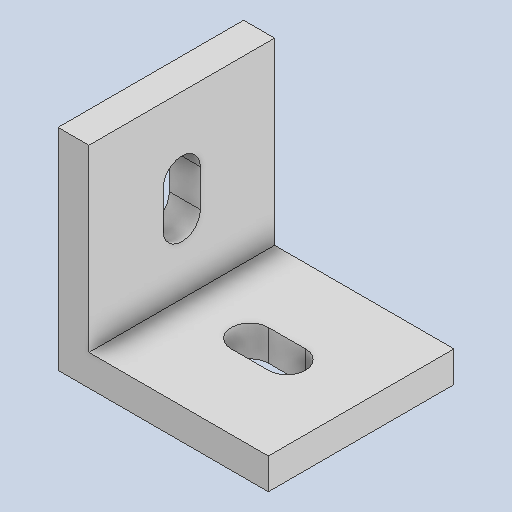
# Autodesk Inventor part: L
Saved by Autodesk Inventor 2025 (Build 290162000, 162)
## iProperties
Created: 2025-09-03
Part Number: L
Material: Generic
Document SubType Name: Modeling
Designer: Pravoslav
Density: 1 g/cm^3
Appearance: Default
Author: Pravoslav
Autodesk Inventor part; units mm, degrees
ref_plane "YZ Plane" through (0, 0, 0) normal (1, 0, 0) x (0, 1, 0)
ref_plane "XZ Plane" through (0, 0, 0) normal (0, 1, 0) x (-1, 0, 0)
ref_plane "XY Plane" through (0, 0, 0) normal (0, 0, 1) x (1, 0, 0)
sketch "Sketch1" plane through (0, 0, 0) normal (0, 1, 0) x (-1, 0, 0)
  line L0 (17, 15) -> (-17, 15)
  line L1 (-17, 15) -> (-17, -15)
  line L2 (-17, -15) -> (17, -15)
  line L3 (17, -15) -> (17, 15)
  line L4 (17, 15) -> (-17, -15) construction
  line L5 (-17, 15) -> (17, -15) construction
  circle A0 centre (-5, 0) radius 3
  circle A1 centre (1, 0) radius 3
  line L6 (1, 3) -> (-5, 3)
  line L7 (1, -3) -> (-5, -3)
  point P0 (0, 0)
  dimension "d0" = 34
  dimension "d1" = 30
  dimension "d2" = 6
  dimension "d3" = 12
  dimension "d4" = 6
  dimension "d5" = 18
  constraints: 16 end point, 4 point on circle, 3 parallel, 2 centre point, 2 horizontal, 2 midpoint, 1 perpendicular, 1 tangent
  measures "d0" distance of L2.end L1.end
  measures "d1" distance of L1.end L0.end
  measures "d2" diameter of A0
  measures "d3" distance from line of L1 A0.centre
  measures "d4" diameter of A1
  measures "d5" distance from line of L1 A1.centre
extrude "Extrusion1" add sketch "Sketch1" along normal blind 5
sketch "Sketch2" plane through (-17, 0, -15) normal (-1, 0, 0) x (0, 0, 1)
  line L0 (30, 0) -> (0, 0) projected
  line L1 (0, 0) -> (30, 0)
  line L2 (30, 0) -> (30, 34)
  line L3 (30, 34) -> (0, 34)
  line L4 (0, 34) -> (0, 0)
  circle A0 centre (15, 16) radius 3
  circle A1 centre (15, 22) radius 3
  line L5 (12, 22) -> (12, 16)
  line L6 (18, 22) -> (18, 16)
  point P0 (15, 0)
  point P1 (15, 0)
  dimension "d8" = 34
  dimension "d9" = 6
  dimension "d10" = 6
  dimension "d11" = 0
  dimension "d12" = 0
  dimension "d13" = 6
  dimension "d15" = 12
  constraints: 12 end point, 4 point on circle, 3 parallel, 2 centre point, 1 horizontal, 1 midpoint, 1 perpendicular, 1 tangent, 1 vertical
  measures "d8" distance of L2.end L1.end
  measures "d9" diameter of A0
  measures "d10" diameter of A1
  measures "d11" horizontal distance of A0.centre A1.centre
  measures "d12" horizontal distance of point (15, 0) A0.centre
  measures "d13" distance of A1.centre A0.centre
  measures "d15" distance from line of L3 A1.centre
extrude "Extrusion2" add sketch "Sketch2" against normal blind 5
body "Solid1"
